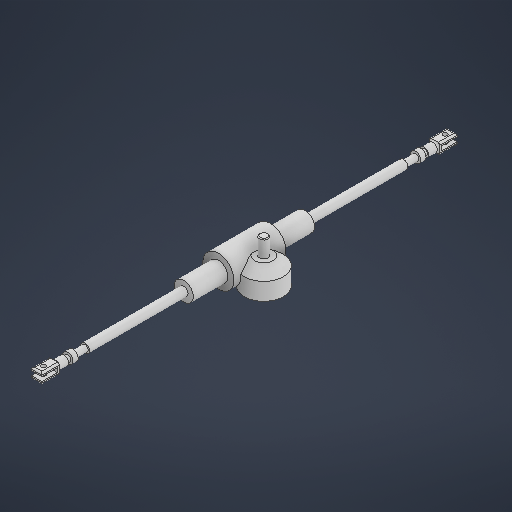
# Autodesk Inventor part: rack
Saved by Autodesk Inventor 2026.2 (Build 302298010, 298A)
## iProperties
Created: 2026-07-06
Part Number: rack
Material: Generic
Document SubType Name: Modeling
Designer: tasle
Density: 1 g/cm^3
Appearance: Default
Author: tasle
Autodesk Inventor part; units mm, degrees
ref_plane "YZ Plane" through (0, 0, 0) normal (1, 0, 0) x (0, 1, 0)
ref_plane "XZ Plane" through (0, 0, 0) normal (0, 1, 0) x (-1, 0, 0)
ref_plane "XY Plane" through (0, 0, 0) normal (0, 0, 1) x (1, 0, 0)
sketch "Sketch1" plane through (0, 0, 0) normal (0, 1, 0) x (-1, 0, 0)
  circle A0 centre (0, 0) radius 22.5
  circle A1 centre (0, 0) radius 5
  dimension "d0" = 45
  dimension "d1" = 10
  constraints: 2 centre point, 2 coincident
  measures "d0" diameter of A0
  measures "d1" diameter of A1
extrude "Extrusion1" add sketch "Sketch1" against normal blind 30 contours A0 | A1
extrude "Extrusion2" add sketch "Sketch1" along normal blind 20 contours A1
chamfer "Chamfer1" distance 12 distance2 10 1 edges at (22.5, 0, 0) measured on face at (22, 0, 0)
sketch "Sketch2" plane through (0, 0, 0) normal (0, 0, 1) x (1, 0, 0)
  circle A0 centre (-22.5, -12) radius 18
  line L0 (5, 20) -> (-5, 20) projected
  line L1 (0, 20) -> (0, -30)
  line L2 (-22.5, -30) -> (22.5, -30) projected
  circle A1 centre (-22.5, -12) radius 11
  point P0 (0, 0)
  dimension "d9" = 36
  dimension "d10" = 18
  dimension "d11" = 22
  constraints: 2 centre point, 2 end point, 2 midpoint, 1 coincident, 1 vertical alignment
  measures "d9" diameter of A0
  measures "d10" distance from line of L2 A0.centre
  measures "d11" diameter of A1
extrude "Extrusion3" add sketch "Sketch2" along normal mid plane 60
extrude "Extrusion4" cut sketch "Sketch2" along normal mid plane 60 contours A1
extrude "Extrusion5" add sketch "Sketch2" along normal mid plane 140 contours A1
sketch "Sketch3" plane through (0, 0, 0) normal (0, 1, 0) x (-1, 0, 0)
  line L0 (33.5, 70) -> (11.5, 70) projected
  line L1 (22.5, 70) -> (22.5, -70)
  line L2 (11.5, -70) -> (33.5, -70) projected
  line L3 (22.5, 220) -> (22.5, -220)
  line L4 (26, 220) -> (19, 220)
  line L5 (19, 220) -> (19, 184)
  line L6 (19, 184) -> (26, 184)
  line L7 (26, 184) -> (26, 220)
  line L8 (27.5, 184) -> (17.5, 184)
  line L9 (17.5, 184) -> (17.5, 70)
  line L10 (17.5, 70) -> (27.5, 70)
  line L11 (27.5, 70) -> (27.5, 184)
  line L12 (28.5, 204) -> (16.5, 204)
  line L13 (16.5, 204) -> (16.5, 198)
  line L14 (16.5, 198) -> (28.5, 198)
  line L15 (28.5, 198) -> (28.5, 204)
  circle A0 centre (0, 0) radius 5 projected
  line L16 (0, 0) -> (61.7987, 0)
  line L17 (33.5, -70) -> (11.5, -70)
  line L18 (26, -220) -> (19, -220)
  line L19 (19, -220) -> (19, -184)
  line L20 (19, -184) -> (26, -184)
  line L21 (26, -184) -> (26, -220)
  line L22 (27.5, -184) -> (17.5, -184)
  line L23 (17.5, -184) -> (17.5, -70)
  line L24 (17.5, -70) -> (27.5, -70)
  line L25 (27.5, -70) -> (27.5, -184)
  line L26 (28.5, -204) -> (16.5, -204)
  line L27 (16.5, -204) -> (16.5, -198)
  line L28 (16.5, -198) -> (28.5, -198)
  line L29 (28.5, -198) -> (28.5, -204)
  point P0 (22.5, 0)
  point P1 (22.5, 184)
  point P2 (22.5, 204)
  point P3 (22.5, -184)
  point P4 (22.5, -204)
  dimension "d18" = 440
  dimension "d19" = 7
  dimension "d20" = 36
  dimension "d21" = 10
  dimension "d22" = 12
  dimension "d23" = 6
  dimension "d24" = 16
  constraints: 56 end point, 14 symmetric about line, 8 midpoint, 6 parallel, 4 horizontal, 4 point on line, 3 perpendicular
  measures "d18" distance of L3.start L3.end
  measures "d19" distance of L6.end L5.end
  measures "d20" distance of L5.end L4.end
  measures "d21" distance of L10.end L9.end
  measures "d22" distance of L14.end L13.end
  measures "d23" distance of L13.end L12.end
  measures "d24" distance between parallel lines of L4 L12
sketch "Sketch4" plane through (-22.5, -12, 70) normal (0, 0, 1) x (1, 0, 0)
  circle A0 centre (0, 0) radius 11 projected
  line L0 (-11, 0) -> (11, 0)
  point P0 (22.5, 12)
  constraints: 2 end point, 2 point on circle, 1 coincident, 1 horizontal
ref_plane "Work Plane1" through (-33.5, -12, 70) normal (0, -1, 0) x (1, 0, 0)
sketch "Sketch5" plane through (-33.5, -12, 70) normal (0, -1, 0) x (1, 0, 0)
  line L0 (22, 0) -> (0, 0) projected
  line L1 (22, 0) -> (0, 0) projected
  line L2 (0, 0) -> (22, 0) projected
  line L3 (7.5, 150) -> (14.5, 150) projected
  line L4 (14.5, 150) -> (14.5, 114) projected
  line L5 (14.5, 114) -> (7.5, 114) projected
  line L6 (7.5, 114) -> (7.5, 150) projected
  line L7 (6, 114) -> (16, 114) projected
  line L8 (16, 114) -> (16, 0) projected
  line L9 (16, 0) -> (6, 0) projected
  line L10 (6, 0) -> (6, 114) projected
  line L11 (5, 134) -> (17, 134) projected
  line L12 (17, 134) -> (17, 128) projected
  line L13 (17, 128) -> (5, 128) projected
  line L14 (5, 128) -> (5, 134) projected
  line L15 (22, 0) -> (0, 0) projected
  line L16 (0, 0) -> (22, 0) projected
  line L17 (0, -140) -> (22, -140) projected
  line L18 (0, -140) -> (22, -140) projected
  line L19 (6, -140) -> (6, -254) projected
  line L20 (16, -254) -> (16, -140) projected
  line L21 (14.5, -254) -> (7.5, -254) projected
  line L22 (6, -254) -> (16, -254) projected
  line L23 (5, -274) -> (17, -274) projected
  line L24 (17, -274) -> (17, -268) projected
  line L25 (5, -268) -> (5, -274) projected
  line L26 (14.5, -290) -> (14.5, -254) projected
  line L27 (7.5, -254) -> (7.5, -290) projected
  line L28 (7.5, -290) -> (14.5, -290) projected
  line L29 (17, -268) -> (5, -268) projected
  line L30 (22, -140) -> (0, -140) projected
  line L31 (16, -140) -> (6, -140) projected
  line L32 (0, -140) -> (22, -140) projected
  line L33 (11, 150) -> (11, -290) projected
  line L34 (6, 0) -> (11, 0)
  line L35 (11, 0) -> (11, -140)
  line L36 (11, -140) -> (6, -140)
  line L37 (6, -140) -> (6, 0)
  point P0 (33.5, -70)
  point P1 (11, 114)
  point P2 (11, 134)
  point P3 (33.5, 0)
  point P4 (11, -254)
  point P5 (11, -274)
  point P6 (7.5, -268)
  point P7 (7.5, -274)
  point P8 (7.5, 134)
  point P9 (7.5, 128)
  constraints: 8 end point, 2 parallel, 1 horizontal, 1 perpendicular, 6 other
revolve "Revolution1" add sketch "Sketch5" angle 360 about axis through (-22.5, -12, 220) along (0, 0, -1) separate body contours L33 L17 L37 L0 | L0 L10 L7 L5 L33 | L33 L21 L22 L19 L17 | L5 L6 L13 L33 | L33 L29 L27 L21 | L13 L6 L11 L33 | L33 L23 L27 L29 | L13 L14 L11 L6 | L11 L6 L3 L33 | L27 L23 L25 L29 | L33 L28 L27 L23
chamfer "Chamfer2" distance 1 angle 45 1 edges at (5, 20, 0)
sketch "Sketch6" plane through (-22.5, -12, 70) normal (0, 0, 1) x (1, 0, 0)
  circle A0 centre (0, 0) radius 5 projected
  circle A1 centre (0, 0) radius 5 projected
  point P0 (22.5, 12)
extrude "Extrusion6" cut sketch "Sketch6" against normal blind 140 bodies 1
sketch "Sketch7" plane through (-22.5, -12, 220) normal (0, 0, 1) x (1, 0, 0)
  circle A0 centre (0, 0) radius 3.5 projected
  circle A1 centre (0, 0) radius 5
  line L0 (-6, 6) -> (6, 6)
  line L1 (6, 6) -> (6, -6)
  line L2 (6, -6) -> (-6, -6)
  line L3 (-6, -6) -> (-6, 6)
  line L4 (-6, 6) -> (6, -6) construction
  line L5 (6, 6) -> (-6, -6) construction
  line L6 (-6, 6) -> (6, 6)
  line L7 (6, 6) -> (6, 2.5)
  line L8 (6, 2.5) -> (-6, 2.5)
  line L9 (-6, 2.5) -> (-6, 6)
  line L10 (-6, -6) -> (6, -6)
  line L11 (6, -6) -> (6, -2.5)
  line L12 (6, -2.5) -> (-6, -2.5)
  line L13 (-6, -2.5) -> (-6, -6)
  point P0 (22.5, 12)
  point P1 (-6, -2.5)
  point P2 (-6, 2.5)
  point P3 (-4.3301, -2.5)
  point P4 (4.3301, -2.5)
  point P5 (4.3301, 2.5)
  point P6 (-4.3301, 2.5)
  dimension "d32" = 10
  dimension "d33" = 12
  dimension "d34" = 12
  dimension "d35" = 3.5
  dimension "d36" = 3.5
  constraints: 28 end point, 6 parallel, 3 horizontal, 3 perpendicular, 2 midpoint, 2 point on line, 1 centre point, 1 coincident
  measures "d32" diameter of A1
  measures "d33" distance of L1.end L2.end
  measures "d34" distance of L0.end L1.end
  measures "d35" distance of L6.end L7.end
  measures "d36" distance of L11.end L10.end
extrude "Extrusion7" add sketch "Sketch7" against normal blind 12 contours A0 L8 A1 L12 | A0 L8 A1 | L12 A1 A0 | A0 L12 A1 L8 bodies 2
extrude "Extrusion8" add sketch "Sketch7" along normal blind 20 contours L8 A0 | A0 L8 A1 | L12 A1 A0 | A0 L12 | A1 L8 L3 L0 L1 | L12 L1 L2 L3 A1 bodies 2
extrude "Extrusion9" add sketch "Sketch7" along normal blind 2 contours A0 L12 L8 | A0 L8 A1 L12 | L8 A0 | A0 L8 A1 | L12 A1 A0 | A0 L12 | A0 L12 A1 L8 | L8 L1 L12 A1 | A1 L12 L3 L8 bodies 2
fillet "Fillet1" radius 2 7 edges at (-16.5, -6, 230) (-28.5, -6, 230) (-16.5, -18, 230) (-28.5, -18, 230) (-27.5, -12, 220) (-22.5, -6, 240) (-22.5, -18, 240)
sketch "Sketch8" plane through (-26.5, -6, 238) normal (0, 1, 0) x (1, 0, 0)
  circle A0 centre (4, 6) radius 2.5
  line L0 (8, 0) -> (0, 0) projected
  point P0 (26.5, 238)
  dimension "d44" = 5
  dimension "d45" = 6
  constraints: 1 centre point
  measures "d44" diameter of A0
  measures "d45" distance from line of L0 A0.centre
extrude "Extrusion10" cut sketch "Sketch8" against normal blind 17.875 bodies 2
mirror "Mirror1" about plane through (0, 0, 0) normal (0, 0, 1) of "Extrusion7", "Extrusion8", "Extrusion9", "Fillet1", "Extrusion10" bodies 2
